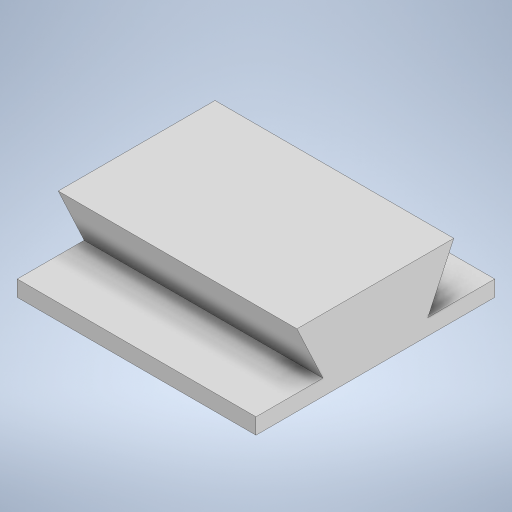
# Autodesk Inventor part: Bottom Sensor Mount
Saved by Autodesk Inventor 2023 (Build 270158000, 158)
## iProperties
Created: 2023-01-24
Part Number: Bottom Sensor Mount
Material: Generic
Document SubType Name: Modeling
Designer: Ahmed Nazir
Density: 1 g/cm^3
Appearance: Default
Author: Ahmed Nazir
Autodesk Inventor part; units mm, degrees
ref_plane "YZ Plane" through (0, 0, 0) normal (1, 0, 0) x (0, 1, 0)
ref_plane "XZ Plane" through (0, 0, 0) normal (0, 1, 0) x (-1, 0, 0)
ref_plane "XY Plane" through (0, 0, 0) normal (0, 0, 1) x (1, 0, 0)
sketch "Sketch1" plane through (0, 0, 0) normal (1, 0, 0) x (0, 1, 0)
  line L0 (0, 0) -> (0, -13.174)
  line L1 (0, -13.174) -> (7, -16.4382)
  line L2 (7, -16.4382) -> (7, 3.2642)
  line L3 (7, 3.2642) -> (0, 0)
  line L4 (0, 8.413) -> (-2, 8.413)
  line L5 (-2, 8.413) -> (-2, -21.587)
  line L6 (-2, -21.587) -> (0, -21.587)
  line L7 (0, -21.587) -> (0, 8.413)
  point P0 (0, -6.587)
  dimension "d0" = 13.174
  dimension "d1" = 65
  dimension "d2" = 65
  dimension "d3" = 7
  dimension "d4" = 2
  dimension "d5" = 30
  constraints: 16 end point, 3 parallel, 2 midpoint, 1 horizontal, 1 perpendicular, 1 vertical
  measures "d0" distance of L0.start L0.end
  measures "d1" angle of L0 L3
  measures "d2" angle of L0 L1
  measures "d3" distance between parallel lines of L2 L0
  measures "d4" distance of L6.end L5.end
  measures "d5" distance of L4.end L5.end
extrude "Extrusion1" add sketch "Sketch1" along normal blind 30
body "Solid1"
